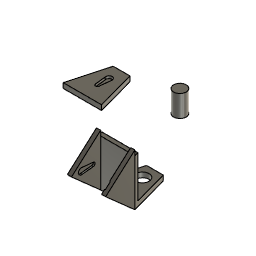
New leg connector (Autodesk Fusion 360 design; units mm, degrees)
Autodesk Fusion 360 part; units mm, degrees
note: some values were not read from the file. Set by a fixed rule: which face or edge a step refers to.
sketch "Sketch1" plane through (0, 0, 0) normal (0, 0, 1) x (1, 0, 0)
  circle A0 centre (0, 5) radius 5
  line L0 (0, 20) -> (-10, 20)
  line L1 (-10, 20) -> (-23, -27)
  line L2 (0, 20) -> (10.087, 20)
  line L3 (10.087, 20) -> (23, -27)
  line L4 (-23, -27) -> (23, -27)
  constraint parallel L0 L2
extrude "Extrude1" add sketch "Sketch1" along normal blind 6 makes body 1
copy_body "CopyPasteBodies1" bodies 1 makes body 2
move_body "Move1" bodies 2 to x (1, 0, 0) y (0, 1, 0) z (0, 0, 1) at (-60, 0, 53)
sketch "Sketch2" plane through (0, 0, 6) normal (0, 0, 1) x (-1, 0, 0)
  circle A0 centre (0, -5) radius 5
  line L0 (-10.087, -20) -> (10, -20)
  line L1 (10, -20) -> (23, 27)
  line L2 (23, 27) -> (-23, 27)
  line L3 (-23, 27) -> (-10.087, -20)
  line L4 (0, 22) -> (21.617, 22)
  line L5 (0, 22) -> (-21.6263, 22)
  constraint coincident L1 L4.end
  constraint coincident L3 L5.end
extrude "Extrude2" add sketch "Sketch2" along normal blind 47 contours L1 L2 L3 L4 L5 bodies 1
sketch "Sketch3" plane through (0, -27, 0) normal (0, -1, 0) x (1, 0, 0)
  line L0 (-23, 0) -> (23, 0)
  line L1 (23, 0) -> (23, 53)
  line L2 (23, 53) -> (-23, 53)
  line L3 (-23, 53) -> (-23, 0)
sketch "Sketch4" plane through (-14.4281, 3.9907, 0) normal (-0.963811, 0.266586, 0) x (-0.266586, -0.963811, 0)
  line L0 (-16.6104, 0) -> (32.1544, 0)
  line L1 (32.1544, 0) -> (32.1544, 53)
  line L2 (32.1544, 53) -> (26.9666, 53)
  line L3 (26.9666, 53) -> (26.9666, 6)
  line L4 (26.9666, 6) -> (-16.6104, 6)
  line L5 (-16.6104, 6) -> (-16.6104, 0)
sketch "Sketch5" plane through (0, 0, 53) normal (0, 0, 1) x (-1, 0, 0)
  line L0 (21.617, 22) -> (23, 27)
  line L1 (23, 27) -> (-23, 27)
  line L2 (-23, 27) -> (-21.6263, 22)
  line L3 (-21.6263, 22) -> (21.617, 22)
  line L4 (-23, 27) -> (-16, 27)
  line L5 (-16, 27) -> (-16, 22)
  line L6 (-16, 22) -> (-21.6263, 22)
  constraint coincident L1.end L2.start
  constraint parallel L1 L4
  constraint coincident L3 L5.end
  constraint perpendicular L3 L5
  constraint coincident L2.end L3.start
  constraint perpendicular L5 L6
extrude "Extrude3" add sketch "Sketch5" along normal blind 6 separate body contours L1 L2 L3 L4 L5 L6 makes body 3
move_body "Move2" bodies 2 to x (1, 0, 0) y (0, 1, 0) z (0, 0, 1) at (0, 0, 15)
sketch "Sketch6" plane through (14.4882, 3.9806, 0) normal (0.964268, 0.264928, 0) x (-0.264928, 0.964268, 0)
  line L0 (-32.1286, 0) -> (16.613, 0)
  line L1 (16.613, 0) -> (16.613, 6)
  line L2 (16.613, 6) -> (-26.9433, 6)
  line L3 (-26.9433, 6) -> (-26.9433, 53)
  line L4 (-26.9433, 53) -> (-32.1286, 53)
  line L5 (-32.1286, 53) -> (-32.1286, 0)
sketch "Sketch7" plane through (0, -27, 26.5) normal (0, -1, 0) x (1, 0, 0)
  line L0 (23, 0) -> (23, -26.5)
  line L1 (23, -26.5) -> (23, 32.5)
  line L2 (23, 32.5) -> (16, 32.5)
  line L3 (16, 32.5) -> (16, -26.5)
  line L4 (16, -26.5) -> (23, -26.5)
  constraint vertical L0
  constraint parallel L0 L1
  constraint perpendicular L1 L2
  constraint perpendicular L2 L3
  constraint perpendicular L0 L4
extrude "Extrude4" add sketch "Sketch7" along normal blind 26 bodies 1 3
sketch "Sketch8" plane through (23, 0, 0) normal (1, 0, 0) x (0, 1, 0)
  line L0 (-27, 0) -> (-27, 59)
  line L1 (-27, 59) -> (-53, 59)
  line L2 (-53, 59) -> (-53, 0)
  line L3 (-53, 0) -> (-27, 0)
  line L4 (-53, 0) -> (-53, 29)
  line L5 (-53, 29) -> (-27, 59)
  line L6 (-53, 29) -> (-27, 0)
  dimension "d14" = 29
  constraint coincident L2.end L3.start
  constraint coincident L2 L4.end
  constraint coincident L0.end L1.start
  constraint coincident L0.start L3.end
  measures "d14" distance of L2.end L4.end
extrude "Extrude5" cut sketch "Sketch8" against normal blind 30 contours L1 L2 L5 bodies 1
sketch "Sketch9" plane through (23, 0, 0) normal (1, 0, 0) x (0, 1, 0)
  line L0 (-27, 59) -> (-53, 29)
  line L1 (-53, 29) -> (-53, 0)
  line L2 (-53, 0) -> (-27, 0)
  line L3 (-27, 0) -> (-27, 59)
  line L4 (-53, 29) -> (-27, 0)
  constraint coincident L0.end L1.start
  constraint coincident L2.end L3.start
extrude "Extrude6" cut sketch "Sketch9" against normal blind 35 contours L1 L2 L4 bodies 1
sketch "Sketch10" plane through (23, 0, 0) normal (1, 0, 0) x (0, 1, 0)
  line L0 (-53, 29) -> (-27, 0)
  line L1 (-27, 0) -> (-27, 59)
  line L2 (-27, 59) -> (-53, 29)
extrude "Extrude7" cut 1 faces at (20.2088, -25.3333, 59) along direction (0, 0, -1) blind 6 on bodies 1 bodies 1
sketch "Sketch11" plane through (0, 0, 53) normal (0, 0, 1) x (-1, 0, 0)
  line L0 (-21.6263, 22) -> (21.617, 22)
  line L1 (21.617, 22) -> (23, 27)
  line L2 (23, 27) -> (-16, 27)
  line L3 (-16, 27) -> (-23, 27)
  line L4 (-23, 27) -> (-21.6263, 22)
  line L5 (23, 27) -> (16, 27)
  line L6 (16, 27) -> (16, 22)
  dimension "d21" = 7
  constraint coincident L1.end L2.start
  constraint parallel L2 L5
  constraint coincident L0 L6.end
  constraint perpendicular L0 L6
  measures "d21" distance of L1.end L5.end
extrude "Extrude8" add sketch "Sketch11" along normal blind 6 contours L0 L1 L2 L5 L6 bodies 1
sketch "Sketch12" plane through (0, -27, 0) normal (0, -1, 0) x (1, 0, 0)
  line L0 (16, 0) -> (16, 53)
  line L1 (16, 53) -> (-16, 53)
  line L2 (-16, 53) -> (-16, 59)
  line L3 (-16, 59) -> (-23, 59)
  line L4 (-23, 59) -> (-23, 0)
  line L5 (-23, 0) -> (16, 0)
  line L6 (-16, 53) -> (-16, 0)
  line L7 (-16, 53) -> (-16, 59)
  constraint coincident L1.end L2.start
  constraint perpendicular L1 L6
  constraint coincident L2.end L3.start
extrude "Extrude9" add sketch "Sketch12" along normal blind 26 contours L2 L3 L4 L5 L6 L7 bodies 1
sketch "Sketch13" plane through (-23, 0, 0) normal (-1, 0, 0) x (0, -1, 0)
  line L0 (27, 59) -> (27, 0)
  line L1 (27, 0) -> (53, 0)
  line L2 (53, 0) -> (53, 59)
  line L3 (53, 59) -> (27, 59)
  line L4 (53, 0) -> (53, 29)
  line L5 (53, 29) -> (27, 0)
  line L6 (53, 29) -> (27, 59)
  dimension "d26" = 29
  constraint coincident L1.end L2.start
  constraint perpendicular L1 L4
  constraint coincident L0.end L1.start
  constraint coincident L0.start L3.end
  measures "d26" distance of L1.end L4.end
extrude "Extrude10" cut sketch "Sketch13" against normal blind 19 contours L2 L3 L6 | L1 L2 L4 L5 bodies 1
extrude "Extrude11" cut 1 faces at (-20.2057, -25.3333, 59) along direction (0, 0, -1) blind 6 on bodies 1 bodies 1
sketch "Sketch14" plane through (0, -27, 26.5) normal (0, -1, 0) x (1, 0, 0)
sketch "Sketch15" plane through (-16, 0, 0) normal (1, 0, 0) x (0, 1, 0)
  line L0 (-27, 53) -> (-27, 59)
  line L1 (-27, 59) -> (-53, 29)
  line L2 (-53, 29) -> (-27, 0)
  line L3 (-27, 0) -> (-27, 53)
sketch "Sketch16" plane through (0, 0, 74) normal (0, 0, 1) x (-1, 0, 0)
  circle A0 centre (60, -5) radius 5
  line L0 (49.913, -20) -> (70, -20)
  line L1 (70, -20) -> (83, 27)
  line L2 (83, 27) -> (37, 27)
  line L3 (37, 27) -> (49.913, -20)
  circle A1 centre (60, -5) radius 5.5
  dimension "d31" = 11
  constraint concentric A0 A1
  measures "d31" diameter of A1
extrude "Extrude12" cut sketch "Sketch16" against normal blind 25 contours A1 bodies 2
sketch "Sketch17" plane through (0, 0, 6) normal (0, 0, 1) x (-1, 0, 0)
  line L0 (21.617, 22) -> (-21.6263, 22)
  line L1 (-21.6263, 22) -> (-10.087, -20)
  line L2 (-10.087, -20) -> (10, -20)
  line L3 (10, -20) -> (21.617, 22)
  circle A0 centre (0, -5) radius 5
  circle A1 centre (0, -5) radius 5.5
  dimension "d34" = 11
  constraint concentric A0 A1
  measures "d34" diameter of A1
extrude "Extrude13" cut sketch "Sketch17" against normal blind 10 contours A1 bodies 1
cylinder "CylinderPrimitive1" add diameter 10 height 60 placed x (1, 0, 0) y (0, 1, 0) z (0, 0, 1) at (-50, 100, 0) separate body makes body 4
sketch "Sketch19" plane through (0, 0, 74) normal (0, 0, 1) x (-1, 0, 0)
  circle A0 centre (60, -5) radius 5.5
  line L0 (49.913, -20) -> (70, -20)
  line L1 (70, -20) -> (83, 27)
  line L2 (83, 27) -> (37, 27)
  line L3 (37, 27) -> (49.913, -20)
  circle A1 centre (60, -5) radius 8
  constraint concentric A0 A1
extrude "Extrude14" cut sketch "Sketch19" against normal blind 25 contours A1 bodies 2
sketch "Sketch20" plane through (0, 0, 6) normal (0, 0, 1) x (-1, 0, 0)
  circle A0 centre (0, -5) radius 5.5
  line L0 (21.617, 22) -> (-21.6263, 22)
  line L1 (-21.6263, 22) -> (-10.087, -20)
  line L2 (-10.087, -20) -> (10, -20)
  line L3 (10, -20) -> (21.617, 22)
  circle A1 centre (0, -5) radius 8
  dimension "d42" = 16
  constraint concentric A0 A1
  measures "d42" diameter of A1
extrude "Extrude15" cut sketch "Sketch20" against normal blind 25 contours A1 bodies 1
move_body "Move3" bodies 2 to x (1, 0, 0) y (0, 1, 0) z (0, 0, 1) at (60, 0, -15)
sketch "Sketch21" plane through (0, 0, 60) normal (0, 0, 1) x (-1, 0, 0)
  circle A0 centre (50, -100) radius 5
  circle A1 centre (50, -100) radius 7.5
  dimension "d45" = 15
  constraint concentric A0 A1
  measures "d45" diameter of A1
extrude "Extrude16" add sketch "Sketch21" against normal blind 60 bodies 4
copy_body "Body->Comp1" bodies 2 removing the originals makes body 5 in component "Component"
copy_body "Body->Comp2" bodies 4 removing the originals makes body 6 in component "Cylinder"
sketch "Sketch22" plane through (80, -40, 59) normal (0, 0, 1) x (-1, 0, 0)
  circle A0 centre (80, -45) radius 8
  line L0 (69.913, -60) -> (90, -60)
  line L1 (90, -60) -> (103, -13)
  line L2 (103, -13) -> (57, -13)
  line L3 (57, -13) -> (69.913, -60)
sketch "Sketch23" plane through (0, 0, 59) normal (0, 0, 1) x (-1, 0, 0)
  circle A0 centre (70, -35) radius 8
  line L0 (59.913, -50) -> (80, -50)
  line L1 (80, -50) -> (93, -3)
  line L2 (93, -3) -> (47, -3)
  line L3 (47, -3) -> (59.913, -50)
  circle A1 centre (70, -35) radius 8
  constraint concentric A0 A1
extrude "Extrude1'" add sketch "Sketch23" against normal blind 6 contours A0 A1 sketch seen with x (1, 0, 0) y (0, 1, 0) z (0, 0, 1) at (70, -30, 0) bodies 5 in component "Component"
sketch "Sketch24" plane through (0, 0, 0) normal (0, 1, 0) x (1, 0, 0)
extrude "Extrude17" add 1 faces at (5.3364, -23.6667, 53) along direction (0, 0, 1) blind 2 on bodies 1 bodies 1
extrude "Extrude18" add 1 faces at (5.3364, -23.6667, 55) along direction (0, 0, 1) blind 1 on bodies 1 bodies 1
extrude "Extrude19" cut sketch "Sketch10" against normal blind 80 bodies 1
sketch "Sketch25" plane through (0, -27, 0) normal (0, -1, 0) x (1, 0, 0)
  line L0 (-23, 0) -> (23, 0)
  line L1 (23, 0) -> (23, 56)
  line L2 (23, 56) -> (-23, 56)
  line L3 (-23, 56) -> (-23, 0)
  line L4 (23, 56) -> (17, 56)
  line L5 (17, 56) -> (17, 0)
  line L6 (23, 56) -> (23, 62)
  line L7 (23, 62) -> (17, 62)
  line L8 (17, 62) -> (17, 56)
  line L9 (0, 56) -> (0, 38.7033)
  line L10 (-17, 62) -> (-17, 56)
  line L11 (-17, 56) -> (-17, 0)
  line L12 (-23, 62) -> (-17, 62)
  line L13 (-23, 56) -> (-23, 62)
  constraint coincident L1.end L2.start
  constraint perpendicular L1 L4
  constraint coincident L0 L5.end
  constraint perpendicular L0 L5
  constraint perpendicular L4 L6
  constraint perpendicular L6 L7
  constraint perpendicular L4 L8
  constraint midpoint L2 L9.start
  constraint perpendicular L2 L9
  constraint symmetric L4.end L9 L10.end
  constraint symmetric L5.end L9 L11.end
  constraint symmetric L1.end L9 L2.end
  constraint symmetric L6.end L9 L12.start
  constraint symmetric L7.end L9 L10.start
extrude "Extrude20" add sketch "Sketch25" along normal blind 28 contours L0 L2 L3 L11 | L2 L10 L12 L13 | L0 L1 L2 L4 L5 | L2 L4 L6 L7 L8 bodies 1
sketch "Sketch26" plane through (23, 0, 0) normal (1, 0, 0) x (0, 1, 0)
  line L0 (-27, 0) -> (-27, 56)
  line L1 (-27, 56) -> (-27, 62)
  line L2 (-27, 62) -> (-55, 62)
  line L3 (-55, 62) -> (-55, 0)
  line L4 (-55, 0) -> (-27, 0)
  line L5 (-55, 31) -> (-27, 62)
  line L6 (-55, 31) -> (-27, 0)
  constraint midpoint L3 L5.start
  constraint coincident L1.end L2.start
  constraint coincident L0.start L4.end
extrude "Extrude21" cut sketch "Sketch26" against normal blind 85 contours L3 L4 L6 | L2 L3 L5 bodies 1
extrude "Extrude1''" cut 1 faces at (-49.1698, 101.2177, 60) along direction (0, 0, -1) blind 40 on bodies 6 bodies 6 in component "Cylinder"
extrude "Extrude2'" add 1 faces at (-49.1698, 101.2177, 20) along direction (0, 0, 1) blind 6 on bodies 6 bodies 6 in component "Cylinder"
sketch "Sketch27" plane through (0, 0, 6) normal (0, 0, 1) x (-1, 0, 0)
  circle A0 centre (0, -5) radius 8
  line L0 (21.617, 22) -> (-21.6263, 22)
  line L1 (-21.6263, 22) -> (-10.087, -20)
  line L2 (-10.087, -20) -> (10, -20)
  line L3 (10, -20) -> (21.617, 22)
  line L4 (0, -5) -> (3, -5)
  line L5 (3, -5) -> (-3, -5)
  line L6 (-3, -5) -> (0, -5)
  line L7 (0, -2) -> (0, -8)
  constraint coincident A0.centre L4.start
  constraint horizontal L4
  constraint parallel L4 L5
  constraint perpendicular L5 L7
sketch "Sketch28" plane through (0, 0, 6) normal (0, 0, 1) x (1, 0, 0)
extrude "Extrude23" cut 1 faces at (17, -36.3333, 29) along direction (1, 0, 0) blind 1 on bodies 1 bodies 1
extrude "Extrude24" cut 1 faces at (-17, -36.3333, 29) along direction (-1, 0, 0) blind 1 on bodies 1 bodies 1
extrude "Extrude2''" cut sketch "Sketch27" against normal blind 36 contours A0 sketch seen with x (1, 0, 0) y (0, 1, 0) z (0, 0, 1) at (70, -30, 0) bodies 5 in component "Component"
sketch "Sketch29" plane through (0, 0, 6) normal (0, 0, 1) x (-1, 0, 0)
  circle A0 centre (0, -5) radius 8
  line L0 (21.617, 22) -> (-21.6263, 22)
  line L1 (-21.6263, 22) -> (-10.087, -20)
  line L2 (-10.087, -20) -> (10, -20)
  line L3 (10, -20) -> (21.617, 22)
sketch "Sketch30" plane through (0, 0, 59) normal (0, 0, 1) x (-1, 0, 0)
  line L0 (59.913, -50) -> (80, -50)
  line L1 (80, -50) -> (93, -3)
  line L2 (93, -3) -> (47, -3)
  line L3 (47, -3) -> (59.913, -50)
  line L4 (73.6153, -33.9952, 0.0021) -> (72.2365, -20.753, 0.0021)
  line L5 (66.3819, -33.9952, 0.0021) -> (67.7607, -20.753, 0.0021)
  arc A0 through (67.7607, -20.753, 0.0021) (69.9986, -18.736, 0.0021) (72.2365, -20.753, 0.0021)
  arc A1 through (73.6153, -33.9952, 0.0021) (69.9986, -38.736, 0.0021) (66.3819, -33.9952, 0.0021)
extrude "Extrude3'" cut sketch "Sketch30" against normal blind 3 contours L4 L5 A0 A1 in plane through (0, 0, 59.0021) normal (0, 0, 1) sketch seen with x (1, 0, 0) y (0, 1, 0) z (0, 0, 1) at (70, -30, 0) bodies 5 in component "Component"
sketch "Sketch36" plane through (0, 0, 59) normal (0, 0, 1) x (-1, 0, 0)
sketch "Sketch37" plane through (0, 0, 59) normal (0, 0, 1) x (1, 0, 0)
extrude "Extrude26" cut 1 faces at (23, -36.3333, 29) along direction (-1, 0, 0) blind 90 on bodies 1 bodies 1
sketch "Sketch38" plane through (0, -27, 0) normal (0, -1, 0) x (1, 0, 0)
  line L0 (-23, 0) -> (23, 0)
  line L1 (23, 0) -> (23, 56)
  line L2 (23, 56) -> (-23, 56)
  line L3 (-23, 56) -> (-23, 0)
  line L4 (23, 0) -> (18, 0)
  line L5 (18, 0) -> (18, 62)
  line L6 (18, 62) -> (23, 62)
  line L7 (23, 62) -> (23, 0)
  line L8 (-23, 0) -> (-18, 0)
  line L9 (-18, 0) -> (-18, 62)
  line L10 (-18, 62) -> (-23, 62)
  line L11 (-23, 62) -> (-23, 0)
  dimension "d96" = 5
  dimension "d97" = 62
  dimension "d98" = 5
  dimension "d99" = 62
  constraint horizontal L4
  constraint vertical L5
  constraint horizontal L6
  constraint vertical L7
  constraint coincident L0.end L1.start
  constraint horizontal L8
  constraint vertical L9
  constraint horizontal L10
  constraint vertical L11
  constraint coincident L0.start L3.end
  measures "d96" distance of L0.end L4.end
  measures "d97" distance of L0.end L6.end
  measures "d98" distance of L0.start L8.end
  measures "d99" distance of L0.start L10.end
extrude "Extrude27" add sketch "Sketch38" along normal blind 35 contours L0 L2 L3 L8 L9 L11 | L2 L9 L10 L11 | L0 L1 L2 L4 L5 L7 | L2 L5 L6 L7 bodies 1
sketch "Sketch39" plane through (23, 0, 0) normal (1, 0, 0) x (0, 1, 0)
  line L0 (-27, 56) -> (-27, 62)
  line L1 (-27, 62) -> (-62, 62)
  line L2 (-62, 62) -> (-62, 0)
  line L3 (-62, 0) -> (-27, 0)
  line L4 (-27, 0) -> (-27, 56)
  line L5 (-62, 31) -> (-27, 62)
  line L6 (-62, 31) -> (-27, 0)
  constraint midpoint L2 L5.start
  constraint coincident L0.end L1.start
  constraint coincident L3.end L4.start
extrude "Extrude28" cut sketch "Sketch39" against normal blind 120 contours L1 L2 L5 | L2 L3 L6 bodies 1
sketch "Sketch40" plane through (-18, 0, 0) normal (1, 0, 0) x (0, 1, 0)
  line L0 (-27, 62) -> (-62, 31)
  line L1 (-62, 31) -> (-27, 0)
  line L2 (-27, 0) -> (-27, 56)
  line L3 (-27, 56) -> (-27, 62)
  line L4 (-49.1216, 34.6457) -> (-35.7641, 33.2376)
  line L5 (-49.1216, 27.3543) -> (-35.7641, 28.7624)
  arc A0 (-35.7641, 28.7624) -> (-35.7641, 33.2376) centre (-36, 31) ccw
  arc A1 (-49.1216, 34.6457) -> (-49.1216, 27.3543) centre (-50, 31) ccw
  constraint tangent L4 A0
  constraint tangent L5 A0
extrude "Extrude29" cut sketch "Sketch40" against normal blind 2 contours L4 L5 A0 A1 bodies 1
sketch "Sketch41" plane through (-18, 0, 0) normal (1, 0, 0) x (0, 1, 0)
  line L0 (-35.7641, 28.7624) -> (-49.1216, 27.3543)
  arc A0 (-49.1216, 34.6457) -> (-49.1216, 27.3543) centre (-50, 31) ccw
  line L1 (-49.1216, 34.6457) -> (-35.7641, 33.2376)
  arc A1 (-35.7641, 28.7624) -> (-35.7641, 33.2376) centre (-36, 31) ccw
  line L2 (-27, 62) -> (-62, 31)
  line L3 (-62, 31) -> (-27, 0)
  line L4 (-27, 0) -> (-27, 56)
  line L5 (-27, 56) -> (-27, 62)
sketch "Sketch42" plane through (18, 0, 0) normal (-1, 0, 0) x (0, -1, 0)
  line L0 (27, 0) -> (62, 31)
  line L1 (62, 31) -> (27, 62)
  line L2 (27, 62) -> (27, 56)
  line L3 (27, 56) -> (27, 0)
  circle A0 centre (50, 31) radius 4
extrude "Extrude30" cut sketch "Sketch42" against normal blind 2 contours A0 bodies 1
sketch "Sketch43" plane through (18, 0, 0) normal (-1, 0, 0) x (0, -1, 0)
  circle A0 centre (50, 31) radius 4
  line L0 (27, 0) -> (62, 31)
  line L1 (62, 31) -> (27, 62)
  line L2 (27, 62) -> (27, 56)
  line L3 (27, 56) -> (27, 0)
  line L4 (50, 31) -> (55.2754, 36.9561)
  line L5 (50, 31) -> (47.0056, 33.6521)
  line L6 (47.0056, 33.6521) -> (52.281, 39.6082)
  line L7 (50, 31) -> (52.9944, 28.3479)
  line L8 (52.9944, 28.3479) -> (58.2697, 34.3039)
  constraint coincident A0.centre L4.start
  constraint coincident L1 L4.end
  constraint perpendicular L1 L4
  constraint coincident A0 L5.end
  constraint perpendicular L4 L5
  constraint coincident L1 L6.end
  constraint tangent A0 L6
  constraint coincident A0 L7.end
  constraint perpendicular L4 L7
  constraint coincident L1 L8.end
  constraint tangent A0 L8
extrude "Extrude31" cut sketch "Sketch43" against normal blind 0.5 contours A0 L1 L4 L6 | A0 L1 L4 L8 bodies 1
extrude "Extrude32" cut 1 faces at (18.5, -54.3939, 35.975) along direction (1, 0, 0) blind 0.3 on bodies 1 bodies 1
sketch "Sketch33" plane through (-18, 0, 0) normal (1, 0, 0) x (0, 1, 0)
  line L0 (-27, 62) -> (-55, 31)
  line L1 (-55, 31) -> (-27, 0)
  line L2 (-27, 0) -> (-27, 56)
  line L3 (-27, 56) -> (-27, 62)
sketch "Sketch34" plane through (-18, 0, 0) normal (1, 0, 0) x (0, 1, 0)
extrude "Extrude25" [suppressed]
sketch "Sketch35" plane through (-18, 0, 0) normal (1, 0, 0) x (0, 1, 0)
  arc A0 (-30.767, 28.7621) -> (-30.767, 33.2379) centre (-31, 31) ccw
  line L0 (-30.767, 28.7621) -> (-44.0092, 27.3833)
  arc A1 (-44.0092, 34.6167) -> (-44.0092, 27.3833) centre (-45, 31) ccw
  line L1 (-44.0092, 34.6167) -> (-30.767, 33.2379)
  line L2 (-27, 62) -> (-55, 31)
  line L3 (-55, 31) -> (-27, 0)
  line L4 (-27, 0) -> (-27, 56)
  line L5 (-27, 56) -> (-27, 62)
sketch "Sketch31" plane through (0, 0, 59) normal (0, 0, 1) x (-1, 0, 0)
  line L0 (72.1944, -20.767) -> (73.5732, -34.0092)
  arc A0 (66.3398, -34.0092) -> (73.5732, -34.0092) centre (69.9565, -35) ccw
  line L1 (66.3398, -34.0092) -> (67.7186, -20.767)
  arc A1 (72.1944, -20.767) -> (67.7186, -20.767) centre (69.9565, -21) ccw
  line L2 (59.913, -50) -> (80, -50)
  line L3 (80, -50) -> (93, -3)
  line L4 (93, -3) -> (47, -3)
  line L5 (47, -3) -> (59.913, -50)
extrude "Extrude22" [suppressed]
sketch "Sketch32" plane through (0, 0, 6) normal (0, 0, 1) x (1, 0, 0)
component "Component" placed x (1, 0, 0) y (0, 1, 0) z (0, 0, 1) at (-70, 30, 0)
component "Cylinder" placed x (1, 0, 0) y (0, 1, 0) z (0, 0, 1) at (0, 0, 0)
named bodies: "Cylinder"
